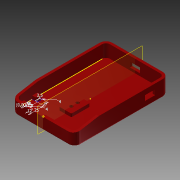
# Autodesk Inventor part: NodeMCU_balance_5kg_base_V0.2
Saved by Autodesk Inventor 2015 (Build 190159000, 159)
## iProperties
Created: 2017-01-21
Part Number: NodeMCU_balance_5kg_base_V0.2
Material: Generic
Document SubType Name: Modeling
Designer: Gordillo
Density: 1 g/cm^3
Appearance: Default
Author: Gordillo
Autodesk Inventor part; units mm, degrees
(part 1 of 2)
ref_plane "XY Plane" through (0, 0, 0) normal (0, 0, 1) x (1, 0, 0)
sketch "Sketch1" plane through (0, 0, 0) normal (0, 0, 1) x (1, 0, 0)
  line L0 (0, 0) -> (0, 200)
  line L1 (0, 0) -> (200, 0) construction
  line L2 (0, 0) -> (100, 0)
  line L3 (0, 0) -> (100, 0) construction
  line L4 (-40, -75) -> (40, -75)
  line L5 (50, -65) -> (50, 65)
  line L6 (40, 75) -> (-40, 75)
  line L7 (-50, 65) -> (-50, -65)
  arc A0 (-40, 75) -> (-50, 65) centre (-40, 65) ccw
  arc A1 (50, 65) -> (40, 75) centre (40, 65) ccw
  arc A2 (-50, -65) -> (-40, -75) centre (-40, -65) ccw
  arc A3 (40, -75) -> (50, -65) centre (40, -65) ccw
  point P0 (50, 75)
  point P1 (50, -75)
  point P2 (-50, 75)
  dimension "d0" = 200
  dimension "d1" = 90
  dimension "d2" = 100
  dimension "d3" = 0
  dimension "ancho_base" = 100
  dimension "largo_base" = 150
  dimension "radio_esquina_base" = 10
  dimension "d7" = 10
  dimension "d8" = 10
  dimension "d9" = 10
  constraints: 16 end point, 8 point on circle, 8 tangent, 6 point on line, 4 centre point, 4 horizontal, 2 equal length, 2 parallel, 1 perpendicular, 1 vertical, 2 other
  measures "d0" distance of L0.start L0.end
  measures "d1" angle of L1 L0
  measures "d2" distance of L0.start L2.end
  measures "d3" distance between parallel lines of L2 L3
  measures "ancho_base" distance of point (50, 75) point (-50, 75)
  measures "largo_base" distance of point (50, -75) point (50, 75)
  measures "radio_esquina_base" radius of A0
  measures "d7" radius of A1
  measures "d8" radius of A2
  measures "d9" radius of A3
extrude "Extrusion1" add sketch "Sketch1" along normal mid plane 5
sketch "Sketch2" plane through (0, 0, 2.5) normal (0, 0, 1) x (1, 0, 0)
  line L0 (-10, -10) -> (10, -10)
  line L1 (10, -10) -> (10, -40)
  line L2 (10, -40) -> (-10, -40)
  line L3 (-10, -40) -> (-10, -10)
  line L4 (0, 0) -> (0, 100)
  line L5 (0, 0) -> (100, 0) construction
  line L6 (-40, -75) -> (40, -75) projected
  dimension "d12" = 20
  dimension "d13" = 30
  dimension "d14" = 100
  dimension "d15" = 90
  dimension "d63" = 35
  constraints: 12 end point, 2 horizontal, 2 parallel, 2 perpendicular, 1 vertical, 1 other
  measures "d12" distance of L1.end L2.end
  measures "d13" distance of L0.end L1.end
  measures "d14" distance of L4.start L4.end
  measures "d15" angle of L5 L4
  measures "d63" distance between parallel lines of L2 L6
extrude "Extrusion2" add sketch "Sketch2" along normal blind 5
fillet "Fillet1" radius 2 4 edges at (-10, -40, 5) (10, -40, 5) (-10, -10, 5) (10, -10, 5)
sketch "Sketch3" plane through (0, 0, 2.5) normal (0, 0, 1) x (1, 0, 0)
  line L0 (40, 75) -> (-40, 75) projected
  arc A0 (-40, 75) -> (-50, 65) centre (-40, 65) ccw projected
  line L1 (-50, 65) -> (-50, -65) projected
  arc A1 (-50, -65) -> (-40, -75) centre (-40, -65) ccw projected
  line L2 (-40, -75) -> (40, -75) projected
  arc A2 (40, -75) -> (50, -65) centre (40, -65) ccw projected
  line L3 (50, -65) -> (50, 65) projected
  arc A3 (50, 65) -> (40, 75) centre (40, 65) ccw projected
  line L4 (-46, -65) -> (-46, 65)
  arc A4 (-40, 71) -> (-46, 65) centre (-40, 65) ccw
  line L5 (-40, 71) -> (40, 71)
  arc A5 (46, 65) -> (40, 71) centre (40, 65) ccw
  line L6 (46, 65) -> (46, -65)
  arc A6 (40, -71) -> (46, -65) centre (40, -65) ccw
  line L7 (40, -71) -> (-40, -71)
  arc A7 (-46, -65) -> (-40, -71) centre (-40, -65) ccw
  point P0 (0, 0)
  dimension "ancho_pared_base" = 4
  constraints: 8 end point, 8 point on circle, 4 centre point, 7 other
  measures "ancho_pared_base" distance between parallel lines of L1 L4
extrude "Extrusion3" add sketch "Sketch3" along normal blind 20
sketch "Sketch4" plane through (0, 0, 7.5) normal (0, 0, 1) x (1, 0, 0)
  circle A0 centre (0, -30) radius 2.5
  line L0 (-10, -38) -> (-10, -12) projected
  line L1 (-10, -25) -> (50, -25)
  line L2 (-10, -25) -> (50, -25) construction
  line L3 (0, 0) -> (0, -100)
  line L4 (40, -71) -> (-40, -71) projected
  line L5 (0, 0) -> (100, 0) construction
  circle A1 centre (0, -20) radius 2.5
  dimension "diametro_agujero_galga" = 5
  dimension "d25" = 60
  dimension "d26" = 360
  dimension "d27" = 100
  dimension "d28" = 90
  dimension "d29" = 5
  constraints: 8 end point, 2 centre point, 2 equal length, 2 horizontal, 2 perpendicular, 1 midpoint, 1 point on line, 1 symmetric about line, 1 other
  measures "diametro_agujero_galga" diameter of A0
  measures "d25" distance of L1.start L1.end
  measures "d27" distance of L3.start L3.end
  measures "d28" angle of L3 L5
  measures "d29" distance from line of L1 A0.centre
extrude "Extrusion4" cut sketch "Sketch4" against normal blind 60
sketch "Sketch5" plane through (0, 0, 7.5) normal (0, 0, 1) x (1, 0, 0)
  line L0 (-6.25, -41.5955) -> (6.25, -41.5955)
  line L1 (6.25, -41.5955) -> (6.25, 33.4045)
  line L2 (6.25, 33.4045) -> (-6.25, 33.4045)
  line L3 (-6.25, 33.4045) -> (-6.25, -41.5955)
  line L4 (8, -10) -> (-8, -10) projected
  line L5 (-8, -40) -> (8, -40) projected
  line L6 (0, 0) -> (0, 100)
  line L7 (0, 0) -> (100, 0) construction
  dimension "anchura_galga" = 12.5
  dimension "largo_galga" = 75
  dimension "d64" = 1.5955
  dimension "d65" = 100
  dimension "d66" = 90
  constraints: 12 end point, 2 horizontal, 2 parallel, 2 perpendicular, 1 vertical, 1 other
  measures "anchura_galga" distance of L2.end L1.end
  measures "largo_galga" distance of L1.end L0.end
  measures "d64" distance between parallel lines of L5 L0
  measures "d65" distance of L6.start L6.end
  measures "d66" angle of L7 L6
extrude "Extrusion5" add sketch "Sketch5" along normal blind 12 separate body
sketch "Sketch6" plane through (0, 0, 19.5) normal (0, 0, 1) x (1, 0, 0)
  circle A0 centre (0, -30) radius 2.5 projected
  circle A1 centre (0, -20) radius 2.5 projected
  point P0 (0, 0)
extrude "Extrusion6" cut sketch "Sketch6" against normal up to surface (12 mm away) bodies 2
ref_plane "Work Plane2" through (-6.25, -4.0955, 7.5) normal (0, -1, 0) x (1, 0, 0)
mirror "Mirror1" about plane through (-6.25, -4.0955, 7.5) normal (0, -1, 0) of "Extrusion6" bodies 2
fillet "Fillet2" radius 2 8 edges at (47.0711, -72.0711, -2.5) (0, -75, -2.5) (-47.0711, -72.0711, -2.5) (-50, 0, -2.5) (-47.0711, 72.0711, -2.5) (0, 75, -2.5) (47.0711, 72.0711, -2.5) (50, 0, -2.5)
ref_plane "Work Plane4" through (-20, -69.9581, 16.5912) normal (0, 0.1736482, -0.9848078) x (-1, 0, 0)
ref_plane "Work Plane3" through (-20, -71, 22.5) normal (0, 0.1736482, -0.9848078) x (-1, 0, 0)
sketch "Sketch8" plane through (-20, -69.9581, 16.5912) normal (0, 0.1736482, -0.9848078) x (-1, 0, 0)
  line L0 (33.2936, -6.6383) -> (-73.3012, -6.6383)
  line L1 (-73.3012, -6.6383) -> (-73.3012, 43.4646)
  line L2 (-73.3012, 43.4646) -> (33.2936, 43.4646)
  line L3 (33.2936, 43.4646) -> (33.2936, -6.6383)
  point P0 (-20, 66.0143)
  constraints: 8 end point, 2 parallel, 1 horizontal, 1 perpendicular
extrude "Extrusion7" cut sketch "Sketch8" against normal blind 12 bodies 1
sketch "Sketch9" plane through (0, 0, 2.5) normal (0, 0, 1) x (1, 0, 0)
  line L0 (-46, 65) -> (-46, -65) projected
  line L1 (-40, -71) -> (40, -71) projected
  line L2 (-46, -38) -> (-42, -38)
  line L3 (-38, -42) -> (-38, -42)
  line L4 (-42, -46) -> (-46, -46)
  line L5 (-46, -46) -> (-46, -38)
  arc A0 (-38, -42) -> (-42, -38) centre (-42, -42) ccw
  arc A1 (-42, -46) -> (-38, -42) centre (-42, -42) ccw
  point P0 (0, 0)
  point P1 (-38, -46)
  point P2 (-38, -38)
  dimension "d47" = 8
  dimension "d48" = 8
  dimension "d49" = 25
  dimension "d167" = 4
  constraints: 8 end point, 5 point on line, 4 point on circle, 4 tangent, 2 centre point, 2 parallel, 1 concentric, 1 horizontal, 1 perpendicular
  measures "d47" distance of point (-38, -46) L4.end
  measures "d48" distance of point (-38, -38) point (-38, -46)
  measures "d49" distance between parallel lines of L1 L4
  measures "d167" radius of A0
extrude "Extrusion8" add sketch "Sketch9" along normal blind 5 bodies 1
sketch "Sketch10" plane through (0, 0, 2.5) normal (0, 0, 1) x (1, 0, 0)
  line L0 (-46, -46) -> (-46, -65) projected
  line L1 (-40, -71) -> (40, -71) projected
  line L2 (-46, -59) -> (-42, -59)
  line L3 (-46, -59) -> (-42, -59) construction
  line L4 (-38, -63) -> (-38, -71)
  line L5 (-40, -71) -> (40, -71) projected
  arc A0 (-46, -65) -> (-40, -71) centre (-40, -65) ccw projected
  line L6 (-46, -46) -> (-46, -65) projected
  arc A1 (-38, -63) -> (-42, -59) centre (-42, -63) ccw
  circle A2 centre (-42, -63) radius 1.15
  circle A3 centre (-41.19, -41.4743) radius 1.25
  circle A4 centre (-41.19, -41.4743) radius 1.25
  point P0 (0, 0)
  point P1 (-38, -59)
  dimension "d52" = 8
  dimension "d53" = 0
  dimension "d168" = 4
  dimension "d169" = 2.3
  dimension "d170" = 2.5
  dimension "d171" = 12
  constraints: 6 end point, 4 centre point, 4 point on line, 2 coincident, 2 horizontal, 2 point on circle, 2 tangent, 1 collinear, 1 concentric, 1 perpendicular
  measures "d52" distance of L2.start point (-38, -59)
  measures "d53" distance between parallel lines of L2 L3
  measures "d168" radius of A1
  measures "d169" diameter of A2
  measures "d170" diameter of A3
  measures "d171" distance between parallel lines of L1 L2
extrude "Extrusion9" add sketch "Sketch10" along normal blind 5 contours L2 A1 L4 L1 A0 L0 | A2 bodies 1
sketch "Sketch12" plane through (-20, -69.9581, 16.5912) normal (0, -0.1736482, 0.9848078) x (1, 0, 0)
  circle A0 centre (62, 29.0257) radius 1.5 projected
  circle A1 centre (62, 5.0346) radius 1.5 projected
  circle A2 centre (-22, 29.0257) radius 1.5 projected
  circle A3 centre (-22, 5.0346) radius 1.5 projected
  line L0 (-30, 5.0346) -> (-30, 34.0277) projected
  ellipse E0 centre (-20, 5.0346) end of major axis (-20, 15.1889) minor radius 10 (-30, 5.0346) -> (-20, -5.1197) ccw projected
  line L1 (60, -5.1197) -> (-20, -5.1197) projected
  ellipse E1 centre (60, 5.0346) end of major axis (60, 15.1889) minor radius 10 (60, -5.1197) -> (70, 5.0346) ccw projected
  line L2 (70, 34.0277) -> (70, 5.0346) projected
  line L3 (66, 34.0277) -> (70, 34.0277) projected
  line L4 (-30, 5.0346) -> (-30, 34.0277) projected
  line L5 (-30, 34.0277) -> (-26, 34.0277) projected
  line L6 (-26, 34.0277) -> (-26, 5.0346) projected
  line L7 (66, 5.0346) -> (66, 34.0277) projected
  line L8 (66, 34.0277) -> (70, 34.0277) projected
  line L9 (70, 34.0277) -> (70, 5.0346) projected
  ellipse E2 centre (60, 5.0346) end of major axis (60, 15.1889) minor radius 10 (60, -5.1197) -> (70, 5.0346) ccw projected
  line L10 (60, -5.1197) -> (-20, -5.1197) projected
  ellipse E3 centre (-20, 5.0346) end of major axis (-20, 15.1889) minor radius 10 (-30, 5.0346) -> (-20, -5.1197) ccw projected
  line L11 (-30, 34.0277) -> (70, 34.0277)
  line L12 (66, 2.4359) -> (66, 130.4609) projected
  ellipse E4 centre (-20, 5.0346) end of major axis (-20, 11.1272) minor radius 6 (-26, 5.0346) -> (-20, -1.058) ccw projected
  line L13 (-20, -1.058) -> (60, -1.058) projected
  ellipse E5 centre (60, 5.0346) end of major axis (60, 11.1272) minor radius 6 (60, -1.058) -> (66, 5.0346) ccw projected
  point P0 (58, 10.4973)
  point P1 (-18, 10.4973)
  point P2 (20, 66.0143)
  point P3 (66, 29.0257)
  constraints: 2 end point, 1 perpendicular, 6 other
extrude "Extrusion11" add sketch "Sketch12" along normal blind 5 separate body contours A0 | A1 | A2 | A3 | L0 L5 L6 E4 L13 E5 L7 L3 L2 E1 L1 E0 | L11 L7 E5 L13 E4 L6
fillet "Fillet3" radius 2 6 edges at (47.0711, -72.9393, 21.1426) (0, -75.8682, 20.6262) (-47.0711, -72.9393, 21.1426) (-50, -51.5919, 24.9067) (50, -51.5919, 24.9067) (0, -37.3156, 27.424)
sketch "Sketch13" plane through (-20, -70.8264, 21.5152) normal (0, -0.1736482, 0.9848078) x (1, 0, 0)
  line L0 (-28, 5.0346) -> (-28, 32.0277) projected
  line L1 (60, -3.1197) -> (-20, -3.1197) projected
  line L2 (68, 32.0277) -> (68, 5.0346) projected
  line L3 (68, 34.0277) -> (-28, 34.0277) projected
  circle A0 centre (62, 29.0257) radius 1.5 projected
  circle A1 centre (62, 5.0346) radius 1.5 projected
  circle A2 centre (-22, 29.0257) radius 1.5 projected
  circle A3 centre (-22, 5.0346) radius 1.5 projected
  line L4 (-28.1214, 5.0346) -> (-28.1214, 32.1491) projected
  line L5 (68.1214, 32.1491) -> (68.1214, 5.0346) projected
  line L6 (60, -3.2411) -> (-20, -3.2411) projected
  line L7 (-28.1214, 32.1491) -> (68.1214, 32.1491) projected
  line L8 (-28, 32.0277) -> (68, 32.0277) projected
  point P0 (20, 66.0143)
  constraints: 4 other
sketch "Sketch16" plane through (-20, -70.8264, 21.5152) normal (0, -0.1736482, 0.9848078) x (1, 0, 0)
  line L0 (68, 32.0277) -> (68, 5.0346) projected
  line L1 (68, 34.0277) -> (-28, 34.0277) projected
  line L2 (29, 30.0277) -> (56, 30.0277)
  line L3 (56, 30.0277) -> (56, 3.0277)
  line L4 (56, 3.0277) -> (29, 3.0277)
  line L5 (29, 3.0277) -> (29, 30.0277)
  point P0 (20, 66.0143)
  dimension "d74" = 27
  dimension "d75" = 27
  dimension "d76" = 12
  dimension "d77" = 4
  constraints: 8 end point, 2 parallel, 1 horizontal, 1 perpendicular
  measures "d74" distance of L3.end L4.end
  measures "d75" distance of L2.end L3.end
  measures "d76" distance between parallel lines of L0 L3
  measures "d77" distance between parallel lines of L1 L2
extrude "Extrusion13" cut sketch "Sketch16" against normal blind 2 bodies 3
sketch "Sketch17" plane through (-20, -70.8264, 21.5152) normal (0, -0.1736482, 0.9848078) x (1, 0, 0)
  line L0 (-28, 5.0346) -> (-28, 32.0277) projected
  line L1 (68, 32.0277) -> (68, 5.0346) projected
  circle A0 centre (-4, 12.0277) radius 6
  line L2 (68, 34.0277) -> (-28, 34.0277) projected
  line L3 (-28, 12.0277) -> (68, 12.0277)
  point P0 (20, 66.0143)
  dimension "d80" = 12
  dimension "d81" = 24
  dimension "d113" = 22
  constraints: 3 point on line, 2 end point, 1 centre point, 1 horizontal
  measures "d80" diameter of A0
  measures "d81" distance from line of L0 A0.centre
  measures "d113" distance between parallel lines of L2 L3
extrude "Extrusion14" cut sketch "Sketch17" against normal up to next bodies 3
sketch "Sketch18" plane through (-20, -70.4791, 19.5456) normal (0, -0.1736482, 0.9848078) x (1, 0, 0)
  line L0 (29, 30.0277) -> (56, 30.0277) projected
  line L1 (29, 3.0277) -> (29, 30.0277) projected
  line L2 (56, 3.0277) -> (29, 3.0277) projected
  line L3 (56, 30.0277) -> (56, 3.0277) projected
  line L4 (42.5, 30.0277) -> (42.5, 3.0277)
  line L5 (29, 16.5277) -> (56, 16.5277)
  circle A0 centre (31, 28.0277) radius 1
  circle A1 centre (54, 28.0277) radius 1
  circle A2 centre (31, 5.0277) radius 1
  circle A3 centre (54, 5.0277) radius 1
  point P0 (20, 66.0143)
  dimension "d84" = 2
  dimension "d85" = 2
  dimension "d86" = 2
  constraints: 4 centre point, 4 end point, 4 midpoint, 3 symmetric about line, 3 other
  measures "d84" diameter of A0
  measures "d85" distance from line of L0 A0.centre
  measures "d86" distance from line of L1 A0.centre
extrude "Extrusion15" cut sketch "Sketch18" against normal up to next contours A0 | A1 | A2 | A3 bodies 3
sketch "Sketch19" plane through (-20, -70.8264, 21.5152) normal (0, -0.1736482, 0.9848078) x (1, 0, 0)
  line L0 (29, 3.0277) -> (29, 30.0277) projected
  line L1 (29, 30.0277) -> (56, 30.0277) projected
  line L2 (56, 30.0277) -> (56, 3.0277) projected
  line L3 (56, 3.0277) -> (29, 3.0277) projected
  line L4 (27.6, 31.4277) -> (27.6, 1.6277)
  line L5 (27.6, 1.6277) -> (57.4, 1.6277)
  line L6 (57.4, 1.6277) -> (57.4, 31.4277)
  line L7 (57.4, 31.4277) -> (27.6, 31.4277)
  point P0 (20, 66.0143)
  dimension "d89" = 1.4
  constraints: 8 end point, 3 other
  measures "d89" distance between parallel lines of L0 L4
extrude "Extrusion16" add sketch "Sketch19" along normal blind 3 separate body contours L0 L1 L2 L3 | L7 L6 L5 L4
fillet "Fillet4" radius 2 4 edges at (22.5, -69.7443, 24.7523) (37.4, -55.0707, 27.3396) (22.5, -40.3971, 29.927) (7.6, -55.0707, 27.3396)
sketch "Sketch20" plane through (-20, -70.4791, 19.5456) normal (0, -0.1736482, 0.9848078) x (1, 0, 0)
  line L0 (29, 30.0277) -> (56, 30.0277) projected
  line L1 (42.5, 30.0277) -> (42.5, 3.0277) projected
  line L2 (29, 16.5277) -> (56, 16.5277) projected
  circle A0 centre (54, 28.0277) radius 1 projected
  circle A1 centre (31, 28.0277) radius 1 projected
  circle A2 centre (31, 5.0277) radius 1 projected
  circle A3 centre (54, 5.0277) radius 1 projected
  circle A4 centre (-4, 12.0277) radius 6 projected
  line L3 (29, 30.0277) -> (29, 3.0277) projected
  line L4 (29, 3.0277) -> (56, 3.0277) projected
  line L5 (56, 3.0277) -> (56, 30.0277) projected
  line L6 (56, 30.0277) -> (29, 30.0277) projected
  line L7 (-30, 5.0346) -> (-30, 34.0277) projected
  line L8 (70, 34.0277) -> (70, 5.0346) projected
  line L9 (60, -5.1197) -> (-20, -5.1197) projected
  line L10 (36.5, 30.0277) -> (48.5, 30.0277)
  line L11 (48.5, 30.0277) -> (48.5, 27.0277)
  line L12 (48.5, 27.0277) -> (36.5, 27.0277)
  line L13 (36.5, 27.0277) -> (36.5, 30.0277)
  line L14 (-30, 34.0277) -> (70, 34.0277) projected
  point P0 (20, 66.0143)
  dimension "d93" = 12
  dimension "d94" = 3
  constraints: 8 end point, 2 parallel, 1 horizontal, 1 perpendicular, 1 point on line, 3 other
  measures "d93" distance of L11.end L12.end
  measures "d94" distance between parallel lines of L0 L12
extrude "Extrusion17" cut sketch "Sketch20" against normal blind 3 contours L0 L1 L12 L13 | L0 L11 L12 L1 bodies 3
fillet "Fillet5" radius 1 3 edges at (16.5, -42.3844, 24.4974) (22.5, -43.8616, 24.2369) (28.5, -42.3844, 24.4974)
sketch "Sketch21" plane through (-20, -71.3473, 24.4696) normal (0, -0.1736482, 0.9848078) x (1, 0, 0)
  line L0 (29.6, 29.4277) -> (55.4, 29.4277) projected
  line L1 (29.6, 3.6277) -> (29.6, 29.4277) projected
  line L2 (55.4, 29.4277) -> (55.4, 3.6277) projected
  line L3 (29.6, 24.4277) -> (55.4, 24.4277)
  line L4 (55.4, 24.4277) -> (55.4, 10.4277)
  line L5 (55.4, 10.4277) -> (29.6, 10.4277)
  line L6 (29.6, 10.4277) -> (29.6, 24.4277)
  point P0 (20, 66.0143)
  dimension "d98" = 14
  dimension "d99" = 5
  constraints: 8 end point, 2 parallel, 2 point on line, 1 horizontal, 1 perpendicular
  measures "d98" distance between parallel lines of L3 L5
  measures "d99" distance between parallel lines of L0 L3
extrude "Extrusion18" cut sketch "Sketch21" against normal up to next contours L3 L2 L5 L1 bodies 4
sketch "Sketch22" plane through (-20, -71.3473, 24.4696) normal (0, -0.1736482, 0.9848078) x (1, 0, 0)
  line L0 (55.4, 29.4277) -> (29.6, 29.4277) projected
  line L1 (29.6, 29.4277) -> (29.6, 24.4277) projected
  line L2 (29.6, 24.4277) -> (29.6, 10.4277) projected
  line L3 (29.6, 10.4277) -> (55.4, 10.4277) projected
  line L4 (55.4, 10.4277) -> (55.4, 24.4277) projected
  line L5 (55.4, 24.4277) -> (55.4, 29.4277) projected
  line L6 (29.6, 10.4277) -> (29.6, 3.6277) projected
  line L7 (29.6, 3.6277) -> (55.4, 3.6277) projected
  line L8 (55.4, 3.6277) -> (55.4, 10.4277) projected
  circle A0 centre (31, 28.0277) radius 1 projected
  circle A1 centre (54, 28.0277) radius 1 projected
  circle A2 centre (54, 5.0277) radius 1 projected
  circle A3 centre (31, 5.0277) radius 1 projected
  line L9 (55.4, 24.4277) -> (29.6, 24.4277) projected
  point P0 (20, 66.0143)
extrude "Extrusion19" cut sketch "Sketch22" against normal up to next contours A0 | A1 | A2 | A3 bodies 4
sketch "Sketch23" plane through (-20, -69.9581, 16.5912) normal (0, 0.1736482, -0.9848078) x (-1, 0, 0)
  circle A0 centre (4, 12.0277) radius 6 projected
  circle A1 centre (4, 12.0277) radius 9
  point P0 (-20, 66.0143)
  dimension "d104" = 3
  constraints: 1 centre point
  measures "d104" radial gap between concentric circles of A0 A1
extrude "Extrusion20" cut sketch "Sketch23" against normal blind 3 bodies 3
sketch "Sketch24" plane through (-24, -58.6341, 21.6342) normal (0, 0.1736482, -0.9848078) x (-1, 0, 0)
  circle A0 centre (0, 0) radius 9 projected
  circle A1 centre (0, 0) radius 8.2
  point P0 (-24, 53.9866)
  dimension "d107" = 0.8
  constraints: 1 centre point
  measures "d107" radial gap between concentric circles of A0 A1
extrude "Extrusion21" add sketch "Sketch24" along normal blind 3.5 separate body contours A1
sketch "Sketch25" plane through (-24, -58.6341, 21.6342) normal (0, -0.1736482, 0.9848078) x (1, 0, 0)
  circle A0 centre (0, 0) radius 6 projected
  circle A1 centre (0, 0) radius 5.5
  point P0 (24, 53.9866)
  dimension "d110" = 0.5
  constraints: 1 centre point
  measures "d110" radial gap between concentric circles of A0 A1
extrude "Extrusion22" add sketch "Sketch25" along normal blind 3.5 contours A1 bodies 5
sketch "Sketch26" plane through (0, 0, -2.5) normal (0, 0, -1) x (-1, 0, 0)
  circle A0 centre (0, -20) radius 2.5 projected
  circle A1 centre (0, -30) radius 2.5 projected
  circle A2 centre (0, -20) radius 5.5
  circle A3 centre (0, -30) radius 5.5
  point P0 (0, 0)
  dimension "d114" = 3
  dimension "d115" = 3
  constraints: 2 centre point
  measures "d114" radial gap between concentric circles of A0 A2
  measures "d115" radial gap between concentric circles of A1 A3
extrude "Extrusion23" cut sketch "Sketch26" against normal blind 3 bodies 1
sketch "Sketch28" plane through (0, 0, 19.5) normal (0, 0, 1) x (1, 0, 0)
  circle A0 centre (0, 21.8091) radius 2.5 projected
  circle A1 centre (0, 11.8091) radius 2.5 projected
  circle A2 centre (0, -20) radius 2.5 projected
  line L0 (-46, -36.4474) -> (-46, 65) projected
  line L1 (46, 65) -> (46, -36.4474) projected
  line L2 (-40, 71) -> (40, 71) projected
  arc A3 (46, 65) -> (40, 71) centre (40, 65) ccw projected
  arc A4 (-40, 71) -> (-46, 65) centre (-40, 65) ccw projected
  line L3 (46, -65) -> (46, 65) projected
  arc A5 (46, 65) -> (40, 71) centre (40, 65) ccw projected
  line L4 (40, 71) -> (-40, 71) projected
  arc A6 (-40, 71) -> (-46, 65) centre (-40, 65) ccw projected
  line L5 (-46, 65) -> (-46, -38) projected
  line L6 (-46, -38) -> (-42, -38) projected
  line L7 (-42, -46) -> (-46, -46) projected
  line L8 (-46, -46) -> (-46, -59) projected
  line L9 (-46, -59) -> (-42, -59) projected
  line L10 (-38, -63) -> (-38, -71) projected
  line L11 (-38, -71) -> (40, -71) projected
  line L12 (10, -12) -> (10, -38) projected
  arc A7 (8, -40) -> (10, -38) centre (8, -38) ccw projected
  line L13 (8, -40) -> (-8, -40) projected
  arc A8 (-10, -38) -> (-8, -40) centre (-8, -38) ccw projected
  line L14 (-10, -38) -> (-10, -12) projected
  arc A9 (-8, -10) -> (-10, -12) centre (-8, -12) ccw projected
  line L15 (-8, -10) -> (8, -10) projected
  arc A10 (10, -12) -> (8, -10) centre (8, -12) ccw projected
  line L16 (48, -37.3156) -> (-48, -37.3156) projected
  line L17 (50, -36.4474) -> (-50, -36.4474) projected
  line L18 (-45, -36.4474) -> (-45, 65)
  arc A11 (-40, 70) -> (-45, 65) centre (-40, 65) ccw
  line L19 (-40, 70) -> (40, 70)
  arc A12 (45, 65) -> (40, 70) centre (40, 65) ccw
  line L20 (45, 65) -> (45, -36.4474)
  line L21 (50, -35.1397) -> (-50, -35.1397)
  line L22 (-45, -35.1397) -> (-45, 65)
  line L23 (-40, 70) -> (40, 70)
  line L24 (45, 65) -> (45, -35.1397)
  line L25 (45, -35.1397) -> (45, 65)
  arc A13 (45, 65) -> (40, 70) centre (40, 65) ccw
  arc A14 (-40, 70) -> (-45, 65) centre (-40, 65) ccw
  arc A15 (-42, -46) -> (-42, -38) centre (-42, -42) ccw projected
  arc A16 (-38, -63) -> (-42, -59) centre (-42, -63) ccw projected
  arc A17 (40, -71) -> (46, -65) centre (40, -65) ccw projected
  point P0 (0, 0)
  dimension "d122" = 1
  constraints: 16 end point, 8 point on circle, 4 centre point, 4 point on line, 3 collinear, 2 concentric, 1 parallel, 1 tangent, 4 other
  measures "d122" distance between parallel lines of L0 L18
extrude "Extrusion25" add sketch "Sketch28" along normal blind 8 separate body contours A2 | L18 A11 L19 A12 L20 L21 L12 A10 L15 A9 L14 | L14 A9 L15 A10 L12 L21
fillet "Fillet6" radius 1 6 edges at (-45, 14.9302, 27.5) (-43.5355, 68.5355, 27.5) (0, 70, 27.5) (43.5355, 68.5355, 27.5) (45, 14.9302, 27.5) (0, -35.1397, 27.5)
sketch "Sketch29" plane through (0, 0, 19.5) normal (0, 0, -1) x (-1, 0, 0)
  line L0 (45, -35.1397) -> (-45, -35.1397) projected
  line L1 (0, 0) -> (30, 0)
  line L2 (6.25, 33.4045) -> (6.25, -41.5955) projected
  line L3 (0, 0) -> (30, 0) construction
  line L4 (0, 0) -> (-30, 0)
  line L5 (0, 0) -> (30, 0) construction
  line L6 (6.25, 33.4045) -> (6.25, -41.5955) projected
  line L7 (-6.25, 33.4045) -> (6.25, 33.4045) projected
  line L8 (-6.25, -41.5955) -> (-6.25, 33.4045) projected
  line L9 (-6.75, -41.5955) -> (-6.75, -35.1397)
  line L10 (0, 0) -> (0, 100) projected
  line L11 (-6.75, 33.9045) -> (6.75, 33.9045)
  line L12 (-6.75, 0) -> (-6.75, 33.9045)
  line L13 (6.75, 0) -> (6.75, 33.9045)
  line L14 (-6.75, 0) -> (-9.75, 0)
  line L15 (-9.75, 0) -> (-9.75, 36.9045)
  line L16 (-9.75, 36.9045) -> (9.75, 36.9045)
  line L17 (9.75, 36.9045) -> (9.75, 0)
  line L18 (9.75, 0) -> (6.75, 0)
  line L19 (-6.75, 0) -> (-9.75, 0)
  dimension "d131" = 30
  dimension "d132" = 0
  dimension "d133" = 30
  dimension "d134" = 180
  dimension "d135" = 0.5
  dimension "d136" = 3
  dimension "d137" = 3
  dimension "d138" = 3
  dimension "d139" = 0.5
  constraints: 28 end point, 5 point on line, 4 collinear, 4 horizontal, 4 perpendicular, 1 symmetric about line
  measures "d131" distance of L1.start L1.end
  measures "d132" distance between parallel lines of L3 L1
  measures "d133" distance of L1.start L4.end
  measures "d134" angle of L4 L5
  measures "d135" distance between parallel lines of L8 L9
  measures "d136" distance of L12.start L14.end
  measures "d137" distance between parallel lines of L13 L17
  measures "d138" distance between parallel lines of L11 L16
  measures "d139" distance between parallel lines of L7 L11
extrude "Extrusion27" add sketch "Sketch29" along normal blind 10 contours L13 L11 L10 L16 L17 L1 | L4 L15 L16 L10 L11 L12 bodies 6
sketch "Sketch30" plane through (0, 0, 19.5) normal (0, 0, -1) x (-1, 0, 0)
  line L0 (-6.75, 0) -> (-9.75, 0) projected
  line L1 (-9.75, 0) -> (-9.75, 36.9045) projected
  line L2 (-9.75, 36.9045) -> (9.75, 36.9045) projected
  line L3 (9.75, 36.9045) -> (9.75, 0) projected
  line L4 (9.75, 0) -> (6.75, 0) projected
  line L5 (6.75, 0) -> (6.75, 33.9045) projected
  line L6 (6.75, 33.9045) -> (-6.75, 33.9045) projected
  line L7 (-6.75, 33.9045) -> (-6.75, 0) projected
  circle A0 centre (0, 11.8091) radius 2.5 projected
  circle A1 centre (0, 21.8091) radius 2.5 projected
  line L8 (45, 65) -> (45, -35.1397) projected
  arc A2 (45, 65) -> (40, 70) centre (40, 65) ccw projected
  line L9 (-40, 70) -> (40, 70) projected
  arc A3 (-40, 70) -> (-45, 65) centre (-40, 65) ccw projected
  line L10 (-45, -35.1397) -> (-45, 65) projected
  line L11 (45, -35.1397) -> (-45, -35.1397) projected
  line L12 (-9.75, 36.9045) -> (-40, 65)
  point P0 (0, 0)
  constraints: 2 end point
ref_plane "Work Plane5" through (9.75, 36.9045, 19.5) normal (0.6805315, -0.7327188, 0) x (0, 0, -1)
sketch "Sketch31" plane through (9.75, 36.9045, 19.5) normal (0.6805315, -0.7327188, 0) x (0, 0, -1)
  line L0 (0, -25.1147) -> (0, 0) projected
  line L1 (10, 0) -> (10, -25.1147) projected
  line L2 (0, 44.9482) -> (1.4456, 12.8188) construction
  line L3 (1.4456, 12.8188) -> (3.0704, 6.6795) construction
  line L4 (3.0704, 6.6795) -> (10, 0) construction
  spline S0 degree 3 poles (0, 44.9482) (1.4456, 12.8188) (3.0704, 6.6795) (10, 0) knots 1 1 1 1 2 2 2 2
  point P0 (19.5, -32.2587)
  point P1 (0, 44.6873)
  constraints: 3 other
sketch "Sketch32" plane through (0, 0, 9.5) normal (0, 0, -1) x (-1, 0, 0)
  line L0 (-6.75, 0) -> (-6.75, 33.9045) projected
  line L1 (-6.75, 33.9045) -> (6.75, 33.9045) projected
  line L2 (6.75, 33.9045) -> (6.75, 0) projected
  line L3 (6.75, 0) -> (9.75, 0) projected
  line L4 (9.75, 0) -> (9.75, 36.9045) projected
  line L5 (9.75, 36.9045) -> (-9.75, 36.9045) projected
  line L6 (-9.75, 36.9045) -> (-9.75, 0) projected
  line L7 (-9.75, 0) -> (-6.75, 0) projected
  line L8 (-9.75, 18.4523) -> (-45, 18.4523)
  line L9 (-45, -35.1397) -> (-45, 65) projected
  point P0 (0, 0)
  constraints: 2 end point, 1 horizontal, 1 midpoint, 1 point on line
sketch "Sketch33" plane through (0, 0, 19.5) normal (0, 0, -1) x (-1, 0, 0)
  line L0 (-6.75, 0) -> (-9.75, 0) projected
  line L1 (-9.75, 0) -> (-9.75, 36.9045) projected
  line L2 (-9.75, 36.9045) -> (9.75, 36.9045) projected
  line L3 (9.75, 36.9045) -> (9.75, 0) projected
  line L4 (9.75, 0) -> (6.75, 0) projected
  line L5 (6.75, 0) -> (6.75, 33.9045) projected
  line L6 (6.75, 33.9045) -> (-6.75, 33.9045) projected
  line L7 (-6.75, 33.9045) -> (-6.75, 0) projected
  circle A0 centre (0, 11.8091) radius 2.5 projected
  circle A1 centre (0, 21.8091) radius 2.5 projected
  line L8 (45, 65) -> (45, -35.1397) projected
  arc A2 (45, 65) -> (40, 70) centre (40, 65) ccw projected
  line L9 (-40, 70) -> (40, 70) projected
  arc A3 (-40, 70) -> (-45, 65) centre (-40, 65) ccw projected
  line L10 (-45, -35.1397) -> (-45, 65) projected
  line L11 (45, -35.1397) -> (-45, -35.1397) projected
  line L12 (-9.75, 18.4523) -> (-45, 18.4523) projected
  point P0 (0, 0)
ref_plane "Work Plane6" through (9.75, 18.4523, 19.5) normal (0, -1, 0) x (0, 0, -1)
sketch "Sketch34" plane through (9.75, 18.4523, 19.5) normal (0, -1, 0) x (0, 0, -1)
  line L0 (0, 35.25) -> (1.2078, 20.0391) construction
  line L1 (1.2078, 20.0391) -> (3.8957, 5.5521) construction
  line L2 (3.8957, 5.5521) -> (10, 0) construction
  spline S0 degree 3 poles (0, 35.25) (1.2078, 20.0391) (3.8957, 5.5521) (10, 0) knots 1 1 1 1 2 2 2 2
  point P0 (19.5, -9.75)
  constraints: 3 other
extrude "Rib1" add sketch "Sketch34" along normal mid plane 24 rib yes fills toward (3.1154, 13.9906) open curves S0
mirror "Mirror3" about plane through (0, 0, 0) normal (1, 0, 0) of "Rib1" bodies 6
sketch "Sketch35" plane through (0, 0, 0) normal (1, 0, 0) x (0, 1, 0)
  line L0 (36.9045, 9.5) -> (43.6693, 17.0471) construction
  line L1 (43.6693, 17.0471) -> (58.5499, 17.0471) construction
  line L2 (58.5499, 17.0471) -> (70, 19.5) construction
  spline S0 degree 3 poles (36.9045, 9.5) (43.6693, 17.0471) (58.5499, 17.0471) (70, 19.5) knots 1 1 1 1 2 2 2 2
  point P0 (0, 0)
  constraints: 3 other
extrude "Rib2" add sketch "Sketch35" along normal mid plane 19 rib yes fills toward (51.6851, 16.4593) open curves S0
sketch "Sketch36" plane through (0, 0, 27.5) normal (0, 0, 1) x (1, 0, 0)
  circle A0 centre (0, 11.8091) radius 2.5 projected
  circle A1 centre (0, 21.8091) radius 2.5 projected
  circle A2 centre (0, 21.8091) radius 4
  circle A3 centre (0, 11.8091) radius 4
  point P0 (0, 0)
  dimension "d154" = 8
  dimension "d155" = 8
  constraints: 2 centre point, 2 coincident
  measures "d154" diameter of A2
  measures "d155" diameter of A3
extrude "Extrusion28" cut sketch "Sketch36" against normal blind 4 bodies 6
sketch "Sketch37" plane through (50, -65, -0.5) normal (1, 0, 0) x (0, 0, -1)
  line L0 (-23, 130) -> (0, 130) projected
  line L1 (-23, 28.5526) -> (-23, 130) projected
  line L2 (-15, 102) -> (-7, 102)
  line L3 (-7, 102) -> (-7, 118)
  line L4 (-7, 118) -> (-15, 118)
  line L5 (-15, 118) -> (-15, 102)
  point P0 (-0.5, 65)
  dimension "d158" = 8
  dimension "d159" = 16
  dimension "d160" = 8
  dimension "d161" = 12
  constraints: 8 end point, 2 parallel, 1 horizontal, 1 perpendicular
  measures "d158" distance of L4.end L3.end
  measures "d159" distance of L3.end L2.end
  measures "d160" distance between parallel lines of L1 L5
  measures "d161" distance between parallel lines of L0 L4
extrude "Extrusion29" cut sketch "Sketch37" against normal up to next bodies 1
sketch "Sketch38" plane through (0, 0, 27.5) normal (0, 0, 1) x (1, 0, 0)
  line L0 (-31.2622, 55.0413) -> (30.7286, 55.0413) construction
  line L1 (30.7286, 55.0413) -> (30.7286, 25.6009) construction
  line L2 (30.7286, 25.6009) -> (-31.2622, 25.6009) construction
  line L3 (-31.2622, 25.6009) -> (-31.2622, 55.0413) construction
  spline S0 degree 2 poles (-23.6619, 51.7695) (-23.6619, 50.3344) (-25.3027, 48.6446) (-26.7525, 48.6446) knots 0 0 0 1 2 2 2
  spline S1 degree 2 poles (-26.7525, 48.6446) (-28.2023, 48.6446) (-29.8431, 50.3344) (-29.8431, 51.7695) knots 0 0 0 1 2 2 2
  spline S2 degree 2 poles (-29.8431, 51.7695) (-29.8431, 53.2193) (-28.2023, 54.8993) (-26.7525, 54.8993) knots 0 0 0 1 2 2 2
  spline S3 degree 2 poles (-26.7525, 54.8993) (-25.3125, 54.8993) (-23.6619, 53.2193) (-23.6619, 51.7695) knots 0 0 0 1 2 2 2
  spline S4 degree 2 poles (-25.7093, 50.2462) (-25.4839, 50.5205) (-25.2684, 51.2699) (-25.2684, 51.7744) knots 0 0 0 1 2 2 2
  spline S5 degree 2 poles (-25.2684, 51.7744) (-25.2684, 52.3132) (-25.5182, 53.0724) (-25.719, 53.3075) knots 0 0 0 1 2 2 2
  spline S6 degree 2 poles (-25.719, 53.3075) (-25.9248, 53.5524) (-26.4586, 53.7679) (-26.7525, 53.7679) knots 0 0 0 1 2 2 2
  spline S7 degree 2 poles (-26.7525, 53.7679) (-27.0464, 53.7679) (-27.5656, 53.5573) (-27.7811, 53.3173) knots 0 0 0 1 2 2 2
  spline S8 degree 2 poles (-27.7811, 53.3173) (-27.9819, 53.092) (-28.2366, 52.2936) (-28.2366, 51.7695) knots 0 0 0 1 2 2 2
  spline S9 degree 2 poles (-28.2366, 51.7695) (-28.2366, 51.2307) (-27.9917, 50.4764) (-27.7909, 50.2413) knots 0 0 0 1 2 2 2
  spline S10 degree 2 poles (-27.7909, 50.2413) (-27.5901, 50.0013) (-27.0464, 49.776) (-26.7525, 49.776) knots 0 0 0 1 2 2 2
  spline S11 degree 2 poles (-26.7525, 49.776) (-26.4537, 49.776) (-25.915, 50.0062) (-25.7093, 50.2462) knots 0 0 0 1 2 2 2
  spline S12 degree 2 poles (-17.8382, 51.0985) (-17.8382, 50.5352) (-18.1811, 49.6193) (-18.4554, 49.3205) knots 0 0 0 1 2 2 2
  spline S13 degree 2 poles (-18.4554, 49.3205) (-18.7493, 49.0071) (-19.479, 48.6838) (-19.9003, 48.6838) knots 0 0 0 1 2 2 2
  spline S14 degree 2 poles (-19.9003, 48.6838) (-20.2823, 48.6838) (-20.8211, 48.8503) (-21.1052, 48.9973) knots 0 0 0 1 2 2 2
  line L4 (-21.1052, 48.9973) -> (-21.1052, 47.1115)
  line L5 (-21.1052, 47.1115) -> (-22.5599, 47.1115)
  line L6 (-22.5599, 47.1115) -> (-22.5599, 53.2977)
  line L7 (-22.5599, 53.2977) -> (-21.1052, 53.2977)
  line L8 (-21.1052, 53.2977) -> (-21.1052, 52.8275)
  spline S15 degree 2 poles (-21.1052, 52.8275) (-20.7721, 53.092) (-20.0766, 53.4201) (-19.6211, 53.4201) knots 0 0 0 1 2 2 2
  spline S16 degree 2 poles (-19.6211, 53.4201) (-18.7737, 53.4201) (-17.8382, 52.1809) (-17.8382, 51.0985) knots 0 0 0 1 2 2 2
  spline S17 degree 2 poles (-19.3321, 51.0642) (-19.3321, 51.7254) (-19.7827, 52.3181) (-20.2676, 52.3181) knots 0 0 0 1 2 2 2
  spline S18 degree 2 poles (-20.2676, 52.3181) (-20.4733, 52.3181) (-20.9093, 52.1956) (-21.1052, 52.0781) knots 0 0 0 1 2 2 2
  line L9 (-21.1052, 52.0781) -> (-21.1052, 49.8054)
  spline S19 degree 2 poles (-21.1052, 49.8054) (-20.9582, 49.7515) (-20.6301, 49.7173) (-20.4684, 49.7173) knots 0 0 0 1 2 2 2
  spline S20 degree 2 poles (-20.4684, 49.7173) (-19.8954, 49.7173) (-19.3321, 50.3883) (-19.3321, 51.0642) knots 0 0 0 1 2 2 2
  line L10 (-12.3329, 50.7654) -> (-15.6586, 50.7654)
  spline S21 degree 2 poles (-15.6586, 50.7654) (-15.6244, 50.2315) (-14.8799, 49.6683) (-14.1501, 49.6683) knots 0 0 0 1 2 2 2
  spline S22 degree 2 poles (-14.1501, 49.6683) (-13.6946, 49.6683) (-12.8276, 49.9964) (-12.5778, 50.1875) knots 0 0 0 1 2 2 2
  line L11 (-12.5778, 50.1875) -> (-12.4162, 50.1875)
  line L12 (-12.4162, 50.1875) -> (-12.4162, 49.0218)
  spline S23 degree 2 poles (-12.4162, 49.0218) (-12.906, 48.8258) (-13.7778, 48.6495) (-14.3068, 48.6495) knots 0 0 0 1 2 2 2
  spline S24 degree 2 poles (-14.3068, 48.6495) (-15.6733, 48.6495) (-17.1231, 49.874) (-17.1231, 51.0103) knots 0 0 0 1 2 2 2
  spline S25 degree 2 poles (-17.1231, 51.0103) (-17.1231, 52.1271) (-15.7468, 53.4397) (-14.5517, 53.4397) knots 0 0 0 1 2 2 2
  spline S26 degree 2 poles (-14.5517, 53.4397) (-13.4448, 53.4397) (-12.3329, 52.323) (-12.3329, 51.2748) knots 0 0 0 1 2 2 2
  line L13 (-12.3329, 51.2748) -> (-12.3329, 50.7654)
  spline S27 degree 2 poles (-13.7778, 51.6177) (-13.7876, 52.0732) (-14.2186, 52.5336) (-14.6693, 52.5336) knots 0 0 0 1 2 2 2
  spline S28 degree 2 poles (-14.6693, 52.5336) (-15.0905, 52.5336) (-15.6293, 52.0977) (-15.6635, 51.6177) knots 0 0 0 1 2 2 2
  line L14 (-15.6635, 51.6177) -> (-13.7778, 51.6177)
  line L15 (-6.7639, 48.772) -> (-8.2186, 48.772)
  line L16 (-8.2186, 48.772) -> (-8.2186, 51.0152)
  spline S29 degree 2 poles (-8.2186, 51.0152) (-8.2186, 51.2895) (-8.2774, 51.8332) (-8.3411, 51.9654) knots 0 0 0 1 2 2 2
  spline S30 degree 2 poles (-8.3411, 51.9654) (-8.4244, 52.1124) (-8.7329, 52.2495) (-9.0121, 52.2495) knots 0 0 0 1 2 2 2
  spline S31 degree 2 poles (-9.0121, 52.2495) (-9.208, 52.2495) (-9.6146, 52.1222) (-9.8546, 51.9801) knots 0 0 0 1 2 2 2
  line L17 (-9.8546, 51.9801) -> (-9.8546, 48.772)
  line L18 (-9.8546, 48.772) -> (-11.3093, 48.772)
  line L19 (-11.3093, 48.772) -> (-11.3093, 53.2977)
  line L20 (-11.3093, 53.2977) -> (-9.8546, 53.2977)
  line L21 (-9.8546, 53.2977) -> (-9.8546, 52.7981)
  spline S32 degree 2 poles (-9.8546, 52.7981) (-9.4676, 53.0969) (-8.7574, 53.4201) (-8.3215, 53.4201) knots 0 0 0 1 2 2 2
  spline S33 degree 2 poles (-8.3215, 53.4201) (-7.5868, 53.4201) (-6.7639, 52.5679) (-6.7639, 51.7156) knots 0 0 0 1 2 2 2
  line L22 (-6.7639, 51.7156) -> (-6.7639, 48.772)
  line L23 (5.7503, 54.772) -> (4.134, 48.772)
  line L24 (4.134, 48.772) -> (2.4197, 48.772)
  line L25 (2.4197, 48.772) -> (1.3471, 52.6805)
  line L26 (1.3471, 52.6805) -> (0.2989, 48.772)
  line L27 (0.2989, 48.772) -> (-1.4154, 48.772)
  line L28 (-1.4154, 48.772) -> (-3.0317, 54.772)
  line L29 (-3.0317, 54.772) -> (-1.4154, 54.772)
  line L30 (-1.4154, 54.772) -> (-0.4946, 50.643)
  line L31 (-0.4946, 50.643) -> (0.6124, 54.772)
  line L32 (0.6124, 54.772) -> (2.1552, 54.772)
  line L33 (2.1552, 54.772) -> (3.2083, 50.643)
  line L34 (3.2083, 50.643) -> (4.1732, 54.772)
  line L35 (4.1732, 54.772) -> (5.7503, 54.772)
  line L36 (11.1577, 50.7654) -> (7.832, 50.7654)
  spline S34 degree 2 poles (7.832, 50.7654) (7.8663, 50.2315) (8.6107, 49.6683) (9.3405, 49.6683) knots 0 0 0 1 2 2 2
  spline S35 degree 2 poles (9.3405, 49.6683) (9.7961, 49.6683) (10.663, 49.9964) (10.9128, 50.1875) knots 0 0 0 1 2 2 2
  line L37 (10.9128, 50.1875) -> (11.0744, 50.1875)
  line L38 (11.0744, 50.1875) -> (11.0744, 49.0218)
  spline S36 degree 2 poles (11.0744, 49.0218) (10.5846, 48.8258) (9.7128, 48.6495) (9.1838, 48.6495) knots 0 0 0 1 2 2 2
  spline S37 degree 2 poles (9.1838, 48.6495) (7.8173, 48.6495) (6.3675, 49.874) (6.3675, 51.0103) knots 0 0 0 1 2 2 2
  spline S38 degree 2 poles (6.3675, 51.0103) (6.3675, 52.1271) (7.7438, 53.4397) (8.9389, 53.4397) knots 0 0 0 1 2 2 2
  spline S39 degree 2 poles (8.9389, 53.4397) (10.0459, 53.4397) (11.1577, 52.323) (11.1577, 51.2748) knots 0 0 0 1 2 2 2
  line L39 (11.1577, 51.2748) -> (11.1577, 50.7654)
  spline S40 degree 2 poles (9.7128, 51.6177) (9.703, 52.0732) (9.272, 52.5336) (8.8214, 52.5336) knots 0 0 0 1 2 2 2
  spline S41 degree 2 poles (8.8214, 52.5336) (8.4001, 52.5336) (7.8614, 52.0977) (7.8271, 51.6177) knots 0 0 0 1 2 2 2
  line L40 (7.8271, 51.6177) -> (9.7128, 51.6177)
  line L41 (13.6361, 48.772) -> (12.1814, 48.772)
  line L42 (12.1814, 48.772) -> (12.1814, 53.2977)
  line L43 (12.1814, 53.2977) -> (13.6361, 53.2977)
  line L44 (13.6361, 53.2977) -> (13.6361, 48.772)
  line L45 (13.6752, 53.9393) -> (12.1422, 53.9393)
  line L46 (12.1422, 53.9393) -> (12.1422, 55.0413)
  line L47 (12.1422, 55.0413) -> (13.6752, 55.0413)
  line L48 (13.6752, 55.0413) -> (13.6752, 53.9393)
  spline S42 degree 2 poles (19.401, 49.2911) (19.401, 48.6544) (19.0385, 47.7826) (18.7103, 47.5377) knots 0 0 0 1 2 2 2
  spline S43 degree 2 poles (18.7103, 47.5377) (18.3871, 47.2879) (17.4663, 47.0675) (16.8834, 47.0675) knots 0 0 0 1 2 2 2
  spline S44 degree 2 poles (16.8834, 47.0675) (16.4132, 47.0675) (15.4973, 47.1801) (15.1642, 47.2634) knots 0 0 0 1 2 2 2
  line L49 (15.1642, 47.2634) -> (15.1642, 48.3948)
  line L50 (15.1642, 48.3948) -> (15.3405, 48.3948)
  spline S45 degree 2 poles (15.3405, 48.3948) (15.605, 48.292) (16.3691, 48.1156) (16.6728, 48.1156) knots 0 0 0 1 2 2 2
  spline S46 degree 2 poles (16.6728, 48.1156) (17.0744, 48.1156) (17.574, 48.2626) (17.7112, 48.3997) knots 0 0 0 1 2 2 2
  spline S47 degree 2 poles (17.7112, 48.3997) (17.8336, 48.532) (17.9463, 48.9336) (17.9463, 49.2128) knots 0 0 0 1 2 2 2
  line L51 (17.9463, 49.2128) -> (17.9463, 49.3009)
  spline S48 degree 2 poles (17.9463, 49.3009) (17.6867, 49.0854) (17.0499, 48.8356) (16.6581, 48.8356) knots 0 0 0 1 2 2 2
  spline S49 degree 2 poles (16.6581, 48.8356) (15.7079, 48.8356) (14.6793, 49.9818) (14.6793, 51.1475) knots 0 0 0 1 2 2 2
  spline S50 degree 2 poles (14.6793, 51.1475) (14.6793, 51.7058) (14.9928, 52.5238) (15.2769, 52.8226) knots 0 0 0 1 2 2 2
  spline S51 degree 2 poles (15.2769, 52.8226) (15.5463, 53.1066) (16.3201, 53.4201) (16.7267, 53.4201) knots 0 0 0 1 2 2 2
  spline S52 degree 2 poles (16.7267, 53.4201) (17.094, 53.4201) (17.6916, 53.2487) (17.9365, 53.092) knots 0 0 0 1 2 2 2
  line L52 (17.9365, 53.092) -> (17.9903, 53.2977)
  line L53 (17.9903, 53.2977) -> (19.401, 53.2977)
  line L54 (19.401, 53.2977) -> (19.401, 49.2911)
  line L55 (17.9463, 50.1973) -> (17.9463, 52.2495)
  spline S53 degree 2 poles (17.9463, 52.2495) (17.8238, 52.3034) (17.4614, 52.3622) (17.3144, 52.3622) knots 0 0 0 1 2 2 2
  spline S54 degree 2 poles (17.3144, 52.3622) (16.7463, 52.3622) (16.1732, 51.7058) (16.1732, 51.1181) knots 0 0 0 1 2 2 2
  spline S55 degree 2 poles (16.1732, 51.1181) (16.1732, 50.4618) (16.6581, 49.9475) (17.1381, 49.9475) knots 0 0 0 1 2 2 2
  spline S56 degree 2 poles (17.1381, 49.9475) (17.3536, 49.9475) (17.7748, 50.0846) (17.9463, 50.1973) knots 0 0 0 1 2 2 2
  line L56 (25.3177, 48.772) -> (23.863, 48.772)
  line L57 (23.863, 48.772) -> (23.863, 51.0152)
  spline S57 degree 2 poles (23.863, 51.0152) (23.863, 51.2895) (23.8042, 51.8332) (23.7405, 51.9654) knots 0 0 0 1 2 2 2
  spline S58 degree 2 poles (23.7405, 51.9654) (23.6573, 52.1124) (23.3487, 52.2495) (23.0695, 52.2495) knots 0 0 0 1 2 2 2
  spline S59 degree 2 poles (23.0695, 52.2495) (22.8736, 52.2495) (22.4671, 52.1222) (22.2271, 51.9801) knots 0 0 0 1 2 2 2
  line L58 (22.2271, 51.9801) -> (22.2271, 48.772)
  line L59 (22.2271, 48.772) -> (20.7724, 48.772)
  line L60 (20.7724, 48.772) -> (20.7724, 55.0413)
  line L61 (20.7724, 55.0413) -> (22.2271, 55.0413)
  line L62 (22.2271, 55.0413) -> (22.2271, 52.7981)
  spline S60 degree 2 poles (22.2271, 52.7981) (22.614, 53.0969) (23.3242, 53.4201) (23.7601, 53.4201) knots 0 0 0 1 2 2 2
  spline S61 degree 2 poles (23.7601, 53.4201) (24.4948, 53.4201) (25.3177, 52.5679) (25.3177, 51.7156) knots 0 0 0 1 2 2 2
  line L63 (25.3177, 51.7156) -> (25.3177, 48.772)
  spline S62 degree 2 poles (29.5446, 48.8111) (29.3095, 48.7524) (28.7854, 48.6838) (28.4083, 48.6838) knots 0 0 0 1 2 2 2
  spline S63 degree 2 poles (28.4083, 48.6838) (27.561, 48.6838) (26.7332, 49.3695) (26.7332, 50.1973) knots 0 0 0 1 2 2 2
  line L64 (26.7332, 50.1973) -> (26.7332, 52.3132)
  line L65 (26.7332, 52.3132) -> (26.1356, 52.3132)
  line L66 (26.1356, 52.3132) -> (26.1356, 53.2977)
  line L67 (26.1356, 53.2977) -> (26.7332, 53.2977)
  line L68 (26.7332, 53.2977) -> (26.7332, 54.5907)
  line L69 (26.7332, 54.5907) -> (28.1879, 54.5907)
  line L70 (28.1879, 54.5907) -> (28.1879, 53.2977)
  line L71 (28.1879, 53.2977) -> (29.5446, 53.2977)
  line L72 (29.5446, 53.2977) -> (29.5446, 52.3132)
  line L73 (29.5446, 52.3132) -> (28.1879, 52.3132)
  line L74 (28.1879, 52.3132) -> (28.1879, 50.7066)
  spline S64 degree 2 poles (28.1879, 50.7066) (28.1879, 50.4715) (28.1977, 50.114) (28.2565, 49.9769) knots 0 0 0 1 2 2 2
  spline S65 degree 2 poles (28.2565, 49.9769) (28.3103, 49.8348) (28.5993, 49.6683) (28.8736, 49.6683) knots 0 0 0 1 2 2 2
  spline S66 degree 2 poles (28.8736, 49.6683) (28.9863, 49.6683) (29.3536, 49.7662) (29.4222, 49.8054) knots 0 0 0 1 2 2 2
  line L75 (29.4222, 49.8054) -> (29.5446, 49.8054)
  line L76 (29.5446, 49.8054) -> (29.5446, 48.8111)
  spline S67 degree 2 poles (-6.9648, 40.6619) (-6.9648, 39.7753) (-8.4684, 38.6684) (-9.7566, 38.6684) knots 0 0 0 1 2 2 2
  spline S68 degree 2 poles (-9.7566, 38.6684) (-10.5011, 38.6684) (-11.608, 38.928) (-12.0929, 39.1337) knots 0 0 0 1 2 2 2
  line L77 (-12.0929, 39.1337) -> (-12.0929, 40.5688)
  line L78 (-12.0929, 40.5688) -> (-11.9215, 40.5688)
  spline S69 degree 2 poles (-11.9215, 40.5688) (-11.4464, 40.1868) (-10.2562, 39.7753) (-9.7076, 39.7753) knots 0 0 0 1 2 2 2
  spline S70 degree 2 poles (-9.7076, 39.7753) (-9.5656, 39.7753) (-9.1101, 39.8243) (-8.9631, 39.8782) knots 0 0 0 1 2 2 2
  spline S71 degree 2 poles (-8.9631, 39.8782) (-8.7868, 39.9517) (-8.5566, 40.1721) (-8.5566, 40.3827) knots 0 0 0 1 2 2 2
  spline S72 degree 2 poles (-8.5566, 40.3827) (-8.5566, 40.5835) (-8.8897, 40.8676) (-9.2129, 40.946) knots 0 0 0 1 2 2 2
  spline S73 degree 2 poles (-9.2129, 40.946) (-9.5509, 41.0243) (-10.3052, 41.1664) (-10.6382, 41.2741) knots 0 0 0 1 2 2 2
  spline S74 degree 2 poles (-10.6382, 41.2741) (-11.3925, 41.519) (-12.0586, 42.3615) (-12.0586, 42.9884) knots 0 0 0 1 2 2 2
  spline S75 degree 2 poles (-12.0586, 42.9884) (-12.0586, 43.826) (-10.555, 44.8839) (-9.3746, 44.8839) knots 0 0 0 1 2 2 2
  spline S76 degree 2 poles (-9.3746, 44.8839) (-8.7819, 44.8839) (-7.626, 44.6537) (-7.2048, 44.4823) knots 0 0 0 1 2 2 2
  line L79 (-7.2048, 44.4823) -> (-7.2048, 43.1011)
  line L80 (-7.2048, 43.1011) -> (-7.3713, 43.1011)
  spline S77 degree 2 poles (-7.3713, 43.1011) (-7.7337, 43.39) (-8.7819, 43.7819) (-9.3305, 43.7819) knots 0 0 0 1 2 2 2
  spline S78 degree 2 poles (-9.3305, 43.7819) (-9.5264, 43.7819) (-9.9084, 43.728) (-10.0848, 43.6545) knots 0 0 0 1 2 2 2
  spline S79 degree 2 poles (-10.0848, 43.6545) (-10.2415, 43.5958) (-10.4668, 43.3509) (-10.4668, 43.1941) knots 0 0 0 1 2 2 2
  spline S80 degree 2 poles (-10.4668, 43.1941) (-10.4668, 42.9541) (-10.1044, 42.6994) (-9.5999, 42.5966) knots 0 0 0 1 2 2 2
  spline S81 degree 2 poles (-9.5999, 42.5966) (-9.2717, 42.528) (-8.6595, 42.4007) (-8.3117, 42.288) knots 0 0 0 1 2 2 2
  spline S82 degree 2 poles (-8.3117, 42.288) (-7.6211, 42.0578) (-6.9648, 41.2839) (-6.9648, 40.6619) knots 0 0 0 1 2 2 2
  spline S83 degree 2 poles (-3.6293, 38.6537) (-4.2219, 38.6537) (-5.2015, 38.9378) (-5.5639, 39.2317) knots 0 0 0 1 2 2 2
  spline S84 degree 2 poles (-5.5639, 39.2317) (-5.9215, 39.5256) (-6.3182, 40.417) (-6.3182, 41.0194) knots 0 0 0 1 2 2 2
  spline S85 degree 2 poles (-6.3182, 41.0194) (-6.3182, 41.6513) (-5.897, 42.5721) (-5.515, 42.8709) knots 0 0 0 1 2 2 2
  spline S86 degree 2 poles (-5.515, 42.8709) (-5.1476, 43.1598) (-4.1925, 43.4243) (-3.6733, 43.4243) knots 0 0 0 1 2 2 2
  spline S87 degree 2 poles (-3.6733, 43.4243) (-3.2129, 43.4243) (-2.4293, 43.2235) (-2.0913, 43.0619) knots 0 0 0 1 2 2 2
  line L81 (-2.0913, 43.0619) -> (-2.0913, 41.8227)
  line L82 (-2.0913, 41.8227) -> (-2.297, 41.8227)
  spline S88 degree 2 poles (-2.297, 41.8227) (-2.3803, 41.8962) (-2.6203, 42.0921) (-2.7917, 42.1851) knots 0 0 0 1 2 2 2
  spline S89 degree 2 poles (-2.7917, 42.1851) (-2.9582, 42.2733) (-3.3501, 42.3909) (-3.6097, 42.3909) knots 0 0 0 1 2 2 2
  spline S90 degree 2 poles (-3.6097, 42.3909) (-4.1925, 42.3909) (-4.8146, 41.6513) (-4.8146, 41.0194) knots 0 0 0 1 2 2 2
  spline S91 degree 2 poles (-4.8146, 41.0194) (-4.8146, 40.3631) (-4.1729, 39.6872) (-3.5901, 39.6872) knots 0 0 0 1 2 2 2
  spline S92 degree 2 poles (-3.5901, 39.6872) (-3.3158, 39.6872) (-2.875, 39.8145) (-2.7329, 39.8978) knots 0 0 0 1 2 2 2
  spline S93 degree 2 poles (-2.7329, 39.8978) (-2.5958, 39.9762) (-2.3852, 40.1574) (-2.297, 40.2407) knots 0 0 0 1 2 2 2
  line L83 (-2.297, 40.2407) -> (-2.0913, 40.2407)
  line L84 (-2.0913, 40.2407) -> (-2.0913, 39.0064)
  spline S94 degree 2 poles (-2.0913, 39.0064) (-2.4341, 38.8447) (-3.1786, 38.6537) (-3.6293, 38.6537) knots 0 0 0 1 2 2 2
  spline S95 degree 2 poles (1.6116, 39.2562) (1.494, 39.168) (1.1463, 38.9182) (0.9944, 38.8447) knots 0 0 0 1 2 2 2
  spline S96 degree 2 poles (0.9944, 38.8447) (0.7789, 38.7468) (0.3234, 38.6537) (0.0491, 38.6537) knots 0 0 0 1 2 2 2
  spline S97 degree 2 poles (0.0491, 38.6537) (-0.5974, 38.6537) (-1.4693, 39.4521) (-1.4693, 40.0741) knots 0 0 0 1 2 2 2
  spline S98 degree 2 poles (-1.4693, 40.0741) (-1.4693, 40.5688) (-1.0235, 41.1958) (-0.617, 41.377) knots 0 0 0 1 2 2 2
  spline S99 degree 2 poles (-0.617, 41.377) (-0.2154, 41.5582) (0.9797, 41.7149) (1.6214, 41.7492) knots 0 0 0 1 2 2 2
  line L85 (1.6214, 41.7492) -> (1.6214, 41.7737)
  spline S100 degree 2 poles (1.6214, 41.7737) (1.6214, 42.1509) (1.0091, 42.4349) (0.4116, 42.4349) knots 0 0 0 1 2 2 2
  spline S101 degree 2 poles (0.4116, 42.4349) (0.054, 42.4349) (-0.7639, 42.1802) (-0.9403, 42.1117) knots 0 0 0 1 2 2 2
  line L86 (-0.9403, 42.1117) -> (-1.0725, 42.1117)
  line L87 (-1.0725, 42.1117) -> (-1.0725, 43.2039)
  spline S102 degree 2 poles (-1.0725, 43.2039) (-0.8423, 43.2627) (0.1912, 43.4292) (0.7152, 43.4292) knots 0 0 0 1 2 2 2
  spline S103 degree 2 poles (0.7152, 43.4292) (1.9495, 43.4292) (3.0516, 42.67) (3.0516, 41.8521) knots 0 0 0 1 2 2 2
  line L88 (3.0516, 41.8521) -> (3.0516, 38.7762)
  line L89 (3.0516, 38.7762) -> (1.6116, 38.7762)
  line L90 (1.6116, 38.7762) -> (1.6116, 39.2562)
  line L91 (1.6116, 39.9566) -> (1.6116, 40.897)
  spline S104 degree 2 poles (1.6116, 40.897) (1.3177, 40.8725) (0.632, 40.7892) (0.4507, 40.7304) knots 0 0 0 1 2 2 2
  spline S105 degree 2 poles (0.4507, 40.7304) (0.2352, 40.6668) (0.005, 40.4023) (0.005, 40.1917) knots 0 0 0 1 2 2 2
  spline S106 degree 2 poles (0.005, 40.1917) (0.005, 40.0496) (0.054, 39.8733) (0.152, 39.7949) knots 0 0 0 1 2 2 2
  spline S107 degree 2 poles (0.152, 39.7949) (0.245, 39.7166) (0.4997, 39.6382) (0.774, 39.6382) knots 0 0 0 1 2 2 2
  spline S108 degree 2 poles (0.774, 39.6382) (0.9944, 39.6382) (1.4401, 39.8145) (1.6116, 39.9566) knots 0 0 0 1 2 2 2
  line L92 (5.8385, 38.7762) -> (4.3838, 38.7762)
  line L93 (4.3838, 38.7762) -> (4.3838, 45.0456)
  line L94 (4.3838, 45.0456) -> (5.8385, 45.0456)
  line L95 (5.8385, 45.0456) -> (5.8385, 38.7762)
  line L96 (11.6622, 40.7696) -> (8.3365, 40.7696)
  spline S109 degree 2 poles (8.3365, 40.7696) (8.3707, 40.2358) (9.1152, 39.6725) (9.845, 39.6725) knots 0 0 0 1 2 2 2
  spline S110 degree 2 poles (9.845, 39.6725) (10.3005, 39.6725) (11.1675, 40.0007) (11.4173, 40.1917) knots 0 0 0 1 2 2 2
  line L97 (11.4173, 40.1917) -> (11.5789, 40.1917)
  line L98 (11.5789, 40.1917) -> (11.5789, 39.026)
  spline S111 degree 2 poles (11.5789, 39.026) (11.0891, 38.83) (10.2173, 38.6537) (9.6883, 38.6537) knots 0 0 0 1 2 2 2
  spline S112 degree 2 poles (9.6883, 38.6537) (8.3218, 38.6537) (6.872, 39.8782) (6.872, 41.0145) knots 0 0 0 1 2 2 2
  spline S113 degree 2 poles (6.872, 41.0145) (6.872, 42.1313) (8.2483, 43.4439) (9.4434, 43.4439) knots 0 0 0 1 2 2 2
  spline S114 degree 2 poles (9.4434, 43.4439) (10.5503, 43.4439) (11.6622, 42.3272) (11.6622, 41.279) knots 0 0 0 1 2 2 2
  line L99 (11.6622, 41.279) -> (11.6622, 40.7696)
  spline S115 degree 2 poles (10.2173, 41.6219) (10.2075, 42.0774) (9.7765, 42.5378) (9.3259, 42.5378) knots 0 0 0 1 2 2 2
  spline S116 degree 2 poles (9.3259, 42.5378) (8.9046, 42.5378) (8.3659, 42.1019) (8.3316, 41.6219) knots 0 0 0 1 2 2 2
  line L100 (8.3316, 41.6219) -> (10.2173, 41.6219)